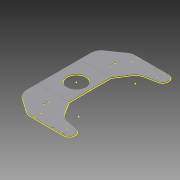
# Autodesk Inventor part: Shell 25083113
Saved by Autodesk Inventor 2013 (Build 170138000, 138)
## iProperties
Created: 2011-09-21
Part Number: Shell 25083113
Document SubType Name: Modeling
Designer: user
Density: 1 g/cm^3
Material: Generic
Author: user
Autodesk Inventor part; units mm, degrees
ref_plane "YZ Plane" through (0, 0, 0) normal (1, 0, 0) x (0, 1, 0)
ref_plane "XZ Plane" through (0, 0, 0) normal (0, 1, 0) x (-1, 0, 0)
ref_plane "XY Plane" through (0, 0, 0) normal (0, 0, 1) x (1, 0, 0)
sketch "Profile" plane through (0, 0, 0) normal (0, 1, 0) x (-1, 0, 0)
  line L0 (-100, 0) -> (-161.7026, -38.5641)
  line L1 (-250, -125) -> (-250, 34.2389)
  line L2 (-240.9616, 62.912) -> (-194.9288, 128.6731)
  line L3 (-153.9672, 150) -> (0, 150)
  line L4 (-195.9806, -129.9029) -> (-184.2316, -71.1582)
  line L5 (-220.4951, -150) -> (-225, -150)
  arc A0 (-161.7026, -38.5641) -> (-184.2316, -71.1582) centre (-135.2026, -80.964) ccw
  arc A1 (-240.9616, 62.912) -> (-250, 34.2389) centre (-200, 34.2389) ccw
  arc A2 (-153.9672, 150) -> (-194.9288, 128.6731) centre (-153.9672, 100) ccw
  arc A3 (-220.4951, -150) -> (-195.9806, -129.9029) centre (-220.4951, -125) ccw
  arc A4 (-250, -125) -> (-225, -150) centre (-225, -125) ccw
  circle A5 centre (-245, -120) radius 2.5
  circle A6 centre (-245, 30) radius 2.5
  line L6 (-163, 47) -> (-173, 47)
  line L7 (-173, 47) -> (-173, 53)
  line L8 (-173, 53) -> (-163, 53)
  line L9 (-163, 53) -> (-163, 47)
  line L10 (-244, -112) -> (-246, -112)
  line L11 (-247, -111) -> (-247, -105)
  line L12 (-246, -104) -> (-244, -104)
  line L13 (-243, -105) -> (-243, -111)
  line L14 (-214, -112) -> (-216, -112)
  line L15 (-217, -111) -> (-217, -105)
  line L16 (-216, -104) -> (-214, -104)
  line L17 (-213, -105) -> (-213, -111)
  arc A7 (-214, -112) -> (-213, -111) centre (-214, -111) ccw
  arc A8 (-217, -111) -> (-216, -112) centre (-216, -111) ccw
  arc A9 (-216, -104) -> (-217, -105) centre (-216, -105) ccw
  arc A10 (-213, -105) -> (-214, -104) centre (-214, -105) ccw
  arc A11 (-243, -105) -> (-244, -104) centre (-244, -105) ccw
  arc A12 (-246, -104) -> (-247, -105) centre (-246, -105) ccw
  arc A13 (-247, -111) -> (-246, -112) centre (-246, -111) ccw
  arc A14 (-244, -112) -> (-243, -111) centre (-244, -111) ccw
  line L18 (-244, 22) -> (-246, 22)
  line L19 (-247, 21) -> (-247, 15)
  line L20 (-246, 14) -> (-244, 14)
  line L21 (-243, 15) -> (-243, 21)
  line L22 (-214, 14) -> (-216, 14)
  line L23 (-217, 15) -> (-217, 21)
  line L24 (-216, 22) -> (-214, 22)
  line L25 (-213, 21) -> (-213, 15)
  arc A15 (-214, 14) -> (-213, 15) centre (-214, 15) ccw
  arc A16 (-217, 15) -> (-216, 14) centre (-216, 15) ccw
  arc A17 (-216, 22) -> (-217, 21) centre (-216, 21) ccw
  arc A18 (-213, 21) -> (-214, 22) centre (-214, 21) ccw
  arc A19 (-243, 21) -> (-244, 22) centre (-244, 21) ccw
  arc A20 (-246, 22) -> (-247, 21) centre (-246, 21) ccw
  arc A21 (-247, 15) -> (-246, 14) centre (-246, 15) ccw
  arc A22 (-244, 14) -> (-243, 15) centre (-244, 15) ccw
  line L26 (100, 0) -> (161.7026, -38.5641)
  line L27 (250, -125) -> (250, 34.2389)
  line L28 (240.9616, 62.912) -> (194.9288, 128.6731)
  line L29 (153.9672, 150) -> (0, 150)
  line L30 (195.9806, -129.9029) -> (184.2316, -71.1582)
  line L31 (220.4951, -150) -> (225, -150)
  arc A23 (184.2316, -71.1582) -> (161.7026, -38.5641) centre (135.2026, -80.964) ccw
  arc A24 (250, 34.2389) -> (240.9616, 62.912) centre (200, 34.2389) ccw
  arc A25 (194.9288, 128.6731) -> (153.9672, 150) centre (153.9672, 100) ccw
  arc A26 (195.9806, -129.9029) -> (220.4951, -150) centre (220.4951, -125) ccw
  arc A27 (225, -150) -> (250, -125) centre (225, -125) ccw
  circle A28 centre (245, -120) radius 2.5
  circle A29 centre (245, 30) radius 2.5
  line L32 (163, 47) -> (173, 47)
  line L33 (173, 47) -> (173, 53)
  line L34 (173, 53) -> (163, 53)
  line L35 (163, 53) -> (163, 47)
  line L36 (244, -112) -> (246, -112)
  line L37 (247, -111) -> (247, -105)
  line L38 (246, -104) -> (244, -104)
  line L39 (243, -105) -> (243, -111)
  line L40 (214, -112) -> (216, -112)
  line L41 (217, -111) -> (217, -105)
  line L42 (216, -104) -> (214, -104)
  line L43 (213, -105) -> (213, -111)
  arc A30 (213, -111) -> (214, -112) centre (214, -111) ccw
  arc A31 (216, -112) -> (217, -111) centre (216, -111) ccw
  arc A32 (217, -105) -> (216, -104) centre (216, -105) ccw
  arc A33 (214, -104) -> (213, -105) centre (214, -105) ccw
  arc A34 (244, -104) -> (243, -105) centre (244, -105) ccw
  arc A35 (247, -105) -> (246, -104) centre (246, -105) ccw
  arc A36 (246, -112) -> (247, -111) centre (246, -111) ccw
  arc A37 (243, -111) -> (244, -112) centre (244, -111) ccw
  line L44 (244, 22) -> (246, 22)
  line L45 (247, 21) -> (247, 15)
  line L46 (246, 14) -> (244, 14)
  line L47 (243, 15) -> (243, 21)
  line L48 (214, 14) -> (216, 14)
  line L49 (217, 15) -> (217, 21)
  line L50 (216, 22) -> (214, 22)
  line L51 (213, 21) -> (213, 15)
  arc A38 (213, 15) -> (214, 14) centre (214, 15) ccw
  arc A39 (216, 14) -> (217, 15) centre (216, 15) ccw
  arc A40 (217, 21) -> (216, 22) centre (216, 21) ccw
  arc A41 (214, 22) -> (213, 21) centre (214, 21) ccw
  arc A42 (244, 22) -> (243, 21) centre (244, 21) ccw
  arc A43 (247, 21) -> (246, 22) centre (246, 21) ccw
  arc A44 (246, 14) -> (247, 15) centre (246, 15) ccw
  arc A45 (243, 15) -> (244, 14) centre (244, 15) ccw
  arc A46 (4.7368, 20.25) -> (-4.7368, 20.25) centre (0, 65) ccw
  line L52 (-100, 0) -> (100, 0)
  line L53 (2.5, 17.7639) -> (2.5, 17.5)
  line L54 (0, 15) -> (0, 15)
  line L55 (-2.5, 17.5) -> (-2.5, 17.7639)
  arc A47 (-2.5, 17.7639) -> (-4.7368, 20.25) centre (-5, 17.7639) ccw
  arc A48 (-2.5, 17.5) -> (0, 15) centre (0, 17.5) ccw
  arc A49 (4.7368, 20.25) -> (2.5, 17.7639) centre (5, 17.7639) ccw
  arc A50 (0, 15) -> (2.5, 17.5) centre (0, 17.5) ccw
  circle A51 centre (-245, -70) radius 2.5
  circle A52 centre (245, -70) radius 2.5
  circle A53 centre (-245, -20) radius 2.5
  circle A54 centre (245, -20) radius 2.5
  line L56 (-153, 47) -> (-143, 47)
  line L57 (-143, 47) -> (-143, 53)
  line L58 (-143, 53) -> (-153, 53)
  line L59 (-153, 53) -> (-153, 47)
  line L60 (153, 47) -> (143, 47)
  line L61 (143, 47) -> (143, 53)
  line L62 (143, 53) -> (153, 53)
  line L63 (153, 53) -> (153, 47)
  point P0 (0, 0)
  point P1 (-180, -50)
  point P2 (-250, -150)
  point P3 (-250, 50)
  point P4 (-180, 150)
  point P5 (-200, -150)
  point P6 (-243, -112)
  point P7 (-247, -104)
  point P8 (-247, -112)
  point P9 (-213, -112)
  point P10 (-217, -104)
  point P11 (-217, -112)
  point P12 (-247, 14)
  point P13 (-247, 22)
  point P14 (-243, 14)
  point P15 (-213, 14)
  point P16 (-217, 14)
  point P17 (-213, 22)
  point P18 (180, -50)
  point P19 (250, -150)
  point P20 (250, 50)
  point P21 (180, 150)
  point P22 (200, -150)
  point P23 (243, -112)
  point P24 (247, -104)
  point P25 (247, -112)
  point P26 (213, -112)
  point P27 (217, -104)
  point P28 (217, -112)
  point P29 (247, 14)
  point P30 (247, 22)
  point P31 (243, 14)
  point P32 (213, 14)
  point P33 (217, 14)
  point P34 (213, 22)
  point P35 (2.5, 15)
  point P36 (-2.5, 15)
  point P37 (-2.5, 20.0695)
  point P38 (2.5, 20.0695)
  dimension "d1" = 80
  dimension "d2" = 50
  dimension "d5" = 200
  dimension "d6" = 100
  dimension "d7" = 70
  dimension "d8" = 180
  dimension "d9" = 20
  dimension "d10" = 100
  dimension "d11" = 50
  dimension "d14" = 50
  dimension "d15" = 25
  dimension "d16" = 5
  dimension "d17" = 5
  dimension "d18" = 150
  dimension "d19" = 5
  dimension "d20" = 5
  dimension "d21" = 30
  dimension "d22" = 10
  dimension "d23" = 6
  dimension "d24" = 97
  dimension "d25" = 73
  dimension "d26" = 4
  dimension "d27" = 8
  dimension "d28" = 8
  dimension "d29" = 7
  dimension "d30" = 4
  dimension "d31" = 8
  dimension "d33" = 8
  dimension "d34" = 1
  dimension "d35" = 8
  dimension "d36" = 4
  dimension "d37" = 7
  dimension "d38" = 8
  dimension "d39" = 4
  dimension "d40" = 8
  dimension "d41" = 30
  dimension "d42" = 8
  dimension "d43" = 1
  dimension "d61" = 30
  dimension "d89" = 8
  dimension "d90" = 4
  dimension "d91" = 8
  dimension "d92" = 4
  dimension "d93" = 30
  dimension "d95" = 7
  dimension "d96" = 5
  dimension "d97" = 8
  dimension "d98" = 4
  dimension "d99" = 8
  dimension "d100" = 4
  dimension "d101" = 30
  dimension "d103" = 7
  dimension "d104" = 5
  dimension "d114" = 90
  dimension "d127" = 97
  dimension "d128" = 6
  dimension "d129" = 10
  dimension "d130" = 73
  dimension "d131" = 65
  dimension "d132" = 100
  dimension "d133" = 200
  dimension "d134" = 5
  dimension "d135" = 2.5
  dimension "d136" = 50
  constraints: 128 end point, 96 point on circle, 74 point on line, 55 centre point, 50 tangent, 20 equal radius, 17 parallel, 8 perpendicular, 7 horizontal
  measures "d1" horizontal distance of point (-180, -50) L0.start
  measures "d2" vertical distance of L0.start point (-180, -50)
  measures "d5" distance of point (-250, -150) point (-250, 50)
  measures "d6" vertical distance of point (-180, 150) point (-250, 50)
  measures "d7" horizontal distance of point (-250, 50) point (-180, 150)
  measures "d8" distance of point (-180, 150) L3.end
  measures "d9" horizontal distance of point (-200, -150) point (-180, -50)
  measures "d10" vertical distance of point (-200, -150) point (-180, -50)
  measures "d11" distance of point (-200, -150) point (-250, -150)
  measures "d14" radius of A0
  measures "d15" radius of A3
  measures "d16" diameter of A5
  measures "d17" diameter of A6
  measures "d18" distance of A6.centre A5.centre
  measures "d19" distance from line of L1 A5.centre
  measures "d20" distance from line of L1 A6.centre
  measures "d21" distance from line of L5 A5.centre
  measures "d22" distance of L7.end L8.end
  measures "d23" distance of L6.end L7.end
  measures "d24" distance between parallel lines of L3 L8
  measures "d25" distance from line of L0.start L7
  measures "d26" distance of point (-243, -112) point (-247, -112)
  measures "d27" distance of point (-247, -112) point (-247, -104)
  measures "d28" distance from line of L10 A5.centre
  measures "d29" distance between parallel lines of L1 L13
  measures "d30" distance of point (-213, -112) point (-217, -112)
  measures "d31" distance of point (-217, -112) point (-217, -104)
  measures "d33" distance from line of L14 A5.centre
  measures "d34" radius of A7
  measures "d35" distance of point (-247, 22) point (-247, 14)
  measures "d36" distance of point (-247, 14) point (-243, 14)
  measures "d37" distance between parallel lines of L1 L21
  measures "d38" distance from line of A6.centre L18
  measures "d39" distance of point (-213, 14) point (-217, 14)
  measures "d40" distance of point (-213, 22) point (-213, 14)
  measures "d41" distance between parallel lines of L19 L23
  measures "d42" distance from line of A6.centre L24
  measures "d43" radius of A15
  measures "d61" distance between parallel lines of L11 L15
  measures "d89" distance between parallel lines of L48 L50
  measures "d90" distance between parallel lines of L49 L51
  measures "d91" distance between parallel lines of L46 L44
  measures "d92" distance between parallel lines of L45 L47
  measures "d93" distance between parallel lines of L45 L49
  measures "d95" distance between parallel lines of L27 L47
  measures "d96" distance from line of L27 A29.centre
  measures "d97" distance between parallel lines of L40 L42
  measures "d98" distance between parallel lines of L41 L43
  measures "d99" distance between parallel lines of L36 L38
  measures "d100" distance between parallel lines of L37 L39
  measures "d101" distance between parallel lines of L37 L41
  measures "d103" distance between parallel lines of L27 L39
  measures "d104" distance from line of L27 A28.centre
  measures "d114" diameter of A46
  measures "d127" distance between parallel lines of L29 L34
  measures "d128" distance of L33.start L33.end
  measures "d129" distance of L32.start L33.start
  measures "d130" distance from line of L26.start L33
  measures "d131" distance from line of A46.centre L52
  measures "d132" distance of L0.start point (0, 0)
  measures "d133" distance of L0.start L26.start
  measures "d134" distance of point (2.5, 15) point (-2.5, 15)
  measures "d135" distance from line of A46.centre L55
  measures "d136" distance from line of A46.centre L54
extrude "Extrusion7" add sketch "Profile" along normal blind 3
sketch "Sketch17" plane through (0, 3, 0) normal (0, 1, 0) x (1, 0, 0)
  arc A0 (-4.7368, -20.25) -> (4.7368, -20.25) centre (0, -65) ccw projected
  line L0 (100, 0) -> (-100, 0) projected
  line L1 (-153.9672, -150) -> (153.9672, -150) projected
  line L2 (-100.25, -10) -> (-99.75, -10)
  line L3 (-99.75, -10) -> (-99.75, -70)
  line L4 (-99.75, -70) -> (-100.25, -70)
  line L5 (-100.25, -70) -> (-100.25, -10)
  line L6 (-100.25, -80) -> (-99.75, -80)
  line L7 (-99.75, -80) -> (-99.75, -140)
  line L8 (-99.75, -140) -> (-100.25, -140)
  line L9 (-100.25, -140) -> (-100.25, -80)
  line L10 (99.75, -10) -> (100.25, -10)
  line L11 (100.25, -10) -> (100.25, -70)
  line L12 (100.25, -70) -> (99.75, -70)
  line L13 (99.75, -70) -> (99.75, -10)
  line L14 (99.75, -80) -> (100.25, -80)
  line L15 (100.25, -80) -> (100.25, -140)
  line L16 (100.25, -140) -> (99.75, -140)
  line L17 (99.75, -140) -> (99.75, -80)
  point P0 (0, 0)
  dimension "d197" = 0.5
  dimension "d199" = 10
  dimension "d200" = 10
  dimension "d201" = 60
  dimension "d202" = 10
  dimension "d203" = 0.5
  dimension "d204" = 99.75
  dimension "d205" = 10
  dimension "d206" = 10
  dimension "d207" = 0.5
  dimension "d208" = 0.5
  dimension "d209" = 60
  dimension "d210" = 99.75
  constraints: 32 end point, 8 parallel, 4 horizontal, 4 perpendicular, 2 collinear
  measures "d197" distance of L2.start L2.end
  measures "d199" distance between parallel lines of L0 L2
  measures "d200" distance between parallel lines of L1 L8
  measures "d201" distance of L4.end L2.start
  measures "d202" distance between parallel lines of L4 L6
  measures "d203" distance of L6.start L6.end
  measures "d204" distance from line of A0.centre L3
  measures "d205" distance between parallel lines of L10 L0
  measures "d206" distance between parallel lines of L14 L12
  measures "d207" distance of L10.start L10.end
  measures "d208" distance of L14.start L14.end
  measures "d209" distance of L10.end L11.end
  measures "d210" distance from line of L13 A0.centre
extrude "Extrusion8" cut sketch "Sketch17" against normal blind 2
sketch "Sketch18" plane through (0, 0, 0) normal (0, -1, 0) x (1, 0, 0)
  arc A0 (4.7368, 20.25) -> (-4.7368, 20.25) centre (0, 65) ccw projected
  arc A1 (4.7368, 20.25) -> (2.5, 17.7639) centre (5, 17.7639) ccw projected
  line L0 (2.5, 17.7639) -> (2.5, 17.5) projected
  arc A2 (-2.5, 17.5) -> (2.5, 17.5) centre (0, 17.5) ccw projected
  line L1 (-2.5, 17.5) -> (-2.5, 17.7639) projected
  arc A3 (-2.5, 17.7639) -> (-4.7368, 20.25) centre (-5, 17.7639) ccw projected
  line L2 (-143, 53) -> (-143, 47) projected
  line L3 (-143, 47) -> (-153, 47) projected
  line L4 (-153, 47) -> (-153, 53) projected
  line L5 (-153, 53) -> (-143, 53) projected
  line L6 (153, 53) -> (153, 47) projected
  line L7 (153, 47) -> (143, 47) projected
  line L8 (143, 47) -> (143, 53) projected
  line L9 (143, 53) -> (153, 53) projected
  line L10 (-163, 53) -> (-163, 47) projected
  line L11 (-163, 47) -> (-173, 47) projected
  line L12 (-173, 47) -> (-173, 53) projected
  line L13 (-173, 53) -> (-163, 53) projected
  line L14 (173, 53) -> (173, 47) projected
  line L15 (173, 47) -> (163, 47) projected
  line L16 (163, 47) -> (163, 53) projected
  line L17 (163, 53) -> (173, 53) projected
  arc A4 (-244, 14) -> (-243, 15) centre (-244, 15) ccw projected
  line L18 (-244, 14) -> (-246, 14) projected
  arc A5 (-247, 15) -> (-246, 14) centre (-246, 15) ccw projected
  line L19 (-247, 15) -> (-247, 21) projected
  arc A6 (-246, 22) -> (-247, 21) centre (-246, 21) ccw projected
  line L20 (-246, 22) -> (-244, 22) projected
  arc A7 (-243, 21) -> (-244, 22) centre (-244, 21) ccw projected
  line L21 (-243, 21) -> (-243, 15) projected
  arc A8 (-213, 21) -> (-214, 22) centre (-214, 21) ccw projected
  line L22 (-213, 21) -> (-213, 15) projected
  arc A9 (-214, 14) -> (-213, 15) centre (-214, 15) ccw projected
  line L23 (-214, 14) -> (-216, 14) projected
  arc A10 (-217, 15) -> (-216, 14) centre (-216, 15) ccw projected
  line L24 (-217, 15) -> (-217, 21) projected
  arc A11 (-216, 22) -> (-217, 21) centre (-216, 21) ccw projected
  line L25 (-216, 22) -> (-214, 22) projected
  arc A12 (-217, -111) -> (-216, -112) centre (-216, -111) ccw projected
  line L26 (-217, -111) -> (-217, -105) projected
  arc A13 (-216, -104) -> (-217, -105) centre (-216, -105) ccw projected
  line L27 (-216, -104) -> (-214, -104) projected
  arc A14 (-213, -105) -> (-214, -104) centre (-214, -105) ccw projected
  line L28 (-213, -105) -> (-213, -111) projected
  arc A15 (-214, -112) -> (-213, -111) centre (-214, -111) ccw projected
  line L29 (-214, -112) -> (-216, -112) projected
  arc A16 (-243, -105) -> (-244, -104) centre (-244, -105) ccw projected
  line L30 (-243, -105) -> (-243, -111) projected
  arc A17 (-244, -112) -> (-243, -111) centre (-244, -111) ccw projected
  line L31 (-244, -112) -> (-246, -112) projected
  arc A18 (-247, -111) -> (-246, -112) centre (-246, -111) ccw projected
  line L32 (-247, -111) -> (-247, -105) projected
  arc A19 (-246, -104) -> (-247, -105) centre (-246, -105) ccw projected
  line L33 (-246, -104) -> (-244, -104) projected
  arc A20 (244, 22) -> (243, 21) centre (244, 21) ccw projected
  line L34 (244, 22) -> (246, 22) projected
  arc A21 (247, 21) -> (246, 22) centre (246, 21) ccw projected
  line L35 (247, 21) -> (247, 15) projected
  arc A22 (246, 14) -> (247, 15) centre (246, 15) ccw projected
  line L36 (246, 14) -> (244, 14) projected
  arc A23 (243, 15) -> (244, 14) centre (244, 15) ccw projected
  line L37 (243, 15) -> (243, 21) projected
  arc A24 (216, 14) -> (217, 15) centre (216, 15) ccw projected
  line L38 (216, 14) -> (214, 14) projected
  arc A25 (213, 15) -> (214, 14) centre (214, 15) ccw projected
  line L39 (213, 15) -> (213, 21) projected
  arc A26 (214, 22) -> (213, 21) centre (214, 21) ccw projected
  line L40 (214, 22) -> (216, 22) projected
  arc A27 (217, 21) -> (216, 22) centre (216, 21) ccw projected
  line L41 (217, 21) -> (217, 15) projected
  arc A28 (244, -104) -> (243, -105) centre (244, -105) ccw projected
  line L42 (244, -104) -> (246, -104) projected
  arc A29 (247, -105) -> (246, -104) centre (246, -105) ccw projected
  line L43 (247, -105) -> (247, -111) projected
  arc A30 (246, -112) -> (247, -111) centre (246, -111) ccw projected
  line L44 (246, -112) -> (244, -112) projected
  arc A31 (243, -111) -> (244, -112) centre (244, -111) ccw projected
  line L45 (243, -111) -> (243, -105) projected
  arc A32 (216, -112) -> (217, -111) centre (216, -111) ccw projected
  line L46 (216, -112) -> (214, -112) projected
  arc A33 (213, -111) -> (214, -112) centre (214, -111) ccw projected
  line L47 (213, -111) -> (213, -105) projected
  arc A34 (214, -104) -> (213, -105) centre (214, -105) ccw projected
  line L48 (214, -104) -> (216, -104) projected
  arc A35 (217, -105) -> (216, -104) centre (216, -105) ccw projected
  line L49 (217, -105) -> (217, -111) projected
  circle A36 centre (-245, -20) radius 2.5 projected
  circle A37 centre (245, -20) radius 2.5 projected
  circle A38 centre (-245, -70) radius 2.5 projected
  circle A39 centre (245, -70) radius 2.5 projected
  circle A40 centre (-245, 30) radius 2.5 projected
  circle A41 centre (-245, -120) radius 2.5 projected
  circle A42 centre (245, 30) radius 2.5 projected
  circle A43 centre (245, -120) radius 2.5 projected
  line L50 (100, 0) -> (161.7026, -38.5641) projected
  arc A44 (184.2316, -71.1582) -> (161.7026, -38.5641) centre (135.2026, -80.964) ccw projected
  line L51 (184.2316, -71.1582) -> (195.9806, -129.9029) projected
  arc A45 (195.9806, -129.9029) -> (220.4951, -150) centre (220.4951, -125) ccw projected
  line L52 (220.4951, -150) -> (225, -150) projected
  arc A46 (225, -150) -> (250, -125) centre (225, -125) ccw projected
  line L53 (250, -125) -> (250, 34.2389) projected
  arc A47 (250, 34.2389) -> (240.9616, 62.912) centre (200, 34.2389) ccw projected
  line L54 (240.9616, 62.912) -> (194.9288, 128.6731) projected
  arc A48 (194.9288, 128.6731) -> (153.9672, 150) centre (153.9672, 100) ccw projected
  line L55 (153.9672, 150) -> (-153.9672, 150) projected
  arc A49 (-153.9672, 150) -> (-194.9288, 128.6731) centre (-153.9672, 100) ccw projected
  line L56 (-194.9288, 128.6731) -> (-240.9616, 62.912) projected
  arc A50 (-240.9616, 62.912) -> (-250, 34.2389) centre (-200, 34.2389) ccw projected
  line L57 (-250, 34.2389) -> (-250, -125) projected
  arc A51 (-250, -125) -> (-225, -150) centre (-225, -125) ccw projected
  line L58 (-225, -150) -> (-220.4951, -150) projected
  arc A52 (-220.4951, -150) -> (-195.9806, -129.9029) centre (-220.4951, -125) ccw projected
  line L59 (-195.9806, -129.9029) -> (-184.2316, -71.1582) projected
  arc A53 (-161.7026, -38.5641) -> (-184.2316, -71.1582) centre (-135.2026, -80.964) ccw projected
  line L60 (-161.7026, -38.5641) -> (-100, 0) projected
  line L61 (-100, 0) -> (100, 0) projected
  line L62 (-100, 0) -> (-100, 150) construction
  line L63 (100, 0) -> (100, 150) construction
  point P0 (0, 0)
  constraints: 4 end point, 2 perpendicular, 2 point on line
body "Solid3"
